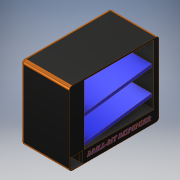
# Autodesk Inventor part: OUTER CASE
Saved by Autodesk Inventor 2019 (Build 230136000, 136)
## iProperties
Created: 2020-03-10
Part Number: OUTER CASE
Material: Gold
Document SubType Name: Modeling
Designer: Hp
Density: 19.3 g/cm^3
Appearance: Metal 1600F Hot
Author: Hp
Autodesk Inventor part; units mm, degrees
ref_plane "YZ Plane" through (0, 0, 0) normal (1, 0, 0) x (0, 1, 0)
ref_plane "XZ Plane" through (0, 0, 0) normal (0, 1, 0) x (-1, 0, 0)
ref_plane "XY Plane" through (0, 0, 0) normal (0, 0, 1) x (1, 0, 0)
sketch "Sketch1" plane through (0, 0, 0) normal (1, 0, 0) x (0, 1, 0)
  line L0 (17.9465, 50) -> (-182.0535, 50)
  line L1 (-182.0535, 50) -> (-182.0535, -300)
  line L2 (-182.0535, -300) -> (17.9465, -300)
  line L3 (17.9465, -300) -> (17.9465, 50)
  point P0 (0, 0)
  dimension "d0" = 200
  dimension "d1" = 350
  constraints: 8 end point, 2 parallel, 1 horizontal, 1 perpendicular
  measures "d0" distance of L2.end L1.end
  measures "d1" distance of L1.end L0.end
extrude "Extrusion1" add sketch "Sketch1" along normal blind 5
sketch "Sketch2" plane through (5, 0, 0) normal (1, 0, 0) x (0, 0, -1)
  circle A0 centre (35, -35.893) radius 14
  line L0 (-50, 17.9465) -> (-50, -182.0535) projected
  line L1 (132.0128, -157.8668) -> (156.8147, -157.8668)
  circle A1 centre (80, -35.893) radius 14
  circle A2 centre (125, -35.893) radius 14
  circle A3 centre (170, -35.893) radius 14
  circle A4 centre (215, -35.893) radius 14
  point P0 (0, 0)
  dimension "d4" = 28
  dimension "d5" = 85
  dimension "d8" = 45
  constraints: 5 centre point, 2 end point, 2 horizontal, 9 other
  measures "d4" diameter of A0
  measures "d8" distance of A0.centre A1.centre
extrude "Extrusion2" cut sketch "Sketch2" against normal blind 1
sketch "Sketch4" plane through (5, 0, 0) normal (1, 0, 0) x (0, 0, -1)
  line L0 (-50, 17.9465) -> (-50, -182.0535) projected
  line L1 (-50, -182.0535) -> (300, -182.0535) projected
  line L2 (-50, 17.9465) -> (0, 17.9465)
  line L3 (0, 17.9465) -> (0, -182.0535)
  line L4 (0, -182.0535) -> (-50, -182.0535)
  line L5 (-50, -182.0535) -> (-50, 17.9465)
  point P0 (0, 0)
  dimension "d17" = 50
  constraints: 8 end point, 2 parallel, 1 horizontal, 1 perpendicular, 1 point on line, 1 other
extrude "Extrusion3" add sketch "Sketch4" along normal blind 150
sketch "Sketch5" plane through (5, 0, 0) normal (1, 0, 0) x (0, 0, -1)
  circle A0 centre (35, -122.0535) radius 14
  line L0 (0, -182.0535) -> (300, -182.0535) projected
  circle A1 centre (80, -122.0535) radius 14
  circle A2 centre (125, -122.0535) radius 14
  circle A3 centre (170, -122.0535) radius 14
  circle A4 centre (215, -122.0535) radius 14
  point P0 (0, 0)
  dimension "d18" = 28
  dimension "d19" = 60
  dimension "d22" = 45
  constraints: 5 centre point, 1 horizontal, 8 other
  measures "d18" diameter of A0
  measures "d19" distance from line of L0 A0.centre
  measures "d22" distance of A0.centre A1.centre
extrude "Extrusion4" cut sketch "Sketch5" against normal blind 2
sketch "Sketch6" plane through (5, 0, 0) normal (1, 0, 0) x (0, 0, -1)
  line L0 (0, -182.0535) -> (300, -182.0535) projected
  line L1 (299.7409, 17.9465) -> (246.5216, 17.9465)
  line L2 (246.5216, 17.9465) -> (246.5216, -182.0535)
  line L3 (246.5216, -182.0535) -> (299.7409, -182.0535)
  line L4 (299.7409, -182.0535) -> (299.7409, 17.9465)
  point P0 (0, 0)
  dimension "d29" = 200
  constraints: 8 end point, 2 parallel, 1 horizontal, 1 perpendicular, 1 point on line
  measures "d29" distance of L3.end L1.start
extrude "Extrusion5" cut sketch "Sketch6" against normal blind 20
sketch "Sketch7" plane through (5, 0, 0) normal (1, 0, 0) x (0, 0, -1)
  line L0 (290.724, 51.1324) -> (325.2992, 51.1324)
  line L1 (325.2992, 51.1324) -> (325.2992, -191.8681)
  line L2 (325.2992, -191.8681) -> (290.724, -191.8681)
  line L3 (290.724, -191.8681) -> (290.724, 51.1324)
  point P0 (0, 0)
  constraints: 8 end point, 2 parallel, 1 horizontal, 1 perpendicular
extrude "Extrusion6" cut sketch "Sketch7" against normal blind 20
sketch "Sketch8" plane through (5, 0, 0) normal (1, 0, 0) x (0, 0, -1)
  line L0 (0, -182.0535) -> (246.5216, -182.0535) projected
  line L1 (246.8963, 18.505) -> (231.8963, 18.505)
  line L2 (231.8963, 18.505) -> (231.8963, -182.0535)
  line L3 (231.8963, -182.0535) -> (246.8963, -182.0535)
  line L4 (246.8963, -182.0535) -> (246.8963, 18.505)
  point P0 (0, 0)
  dimension "d34" = 15
  constraints: 8 end point, 2 parallel, 1 horizontal, 1 perpendicular, 1 point on line
  measures "d34" distance of L3.end L2.end
extrude "Extrusion7" add sketch "Sketch8" along normal blind 150
sketch "Sketch9" plane through (5, -182.0535, 0) normal (0, 0, -1) x (-1, 0, 0)
  point P0 (5, 182.0535)
sketch "Sketch10" plane through (5, 0, 0) normal (1, 0, 0) x (0, 0, -1)
  line L0 (0, -182.0535) -> (0, 17.9465) projected
  line L1 (0, -85.1802) -> (231.8963, -53.9271)
  line L2 (231.8963, -182.0535) -> (231.8963, 17.9465) projected
  line L3 (231.8963, -53.9271) -> (231.8963, -63.9271)
  line L4 (0, -85.1802) -> (0, -95.1802)
  line L5 (0, -95.1802) -> (231.8963, -63.9271)
  line L6 (0, -170.1802) -> (231.8963, -138.9271)
  line L7 (0, -180.1802) -> (231.8963, -148.9271)
  line L8 (0, -170.1802) -> (0, -180.1802)
  line L9 (231.8963, -138.9271) -> (231.8963, -148.9271)
  point P0 (0, 0)
  dimension "d37" = 10
  dimension "d38" = 10
  dimension "d41" = 85
  constraints: 16 end point, 4 point on line, 1 vertical, 8 other
  measures "d37" distance of L1.end L3.end
  measures "d38" distance of L1.start L4.end
  measures "d41" distance of L1.start L6.start
extrude "Extrusion8" add sketch "Sketch10" along normal blind 150 contours L0 L6 L2 L7 | L0 L1 L2 L5
sketch "Sketch11" plane through (0, -182.0535, 50) normal (0, -1, 0) x (1, 0, 0)
  line L0 (150.9028, -4.3641) -> (4.8678, -4.3641)
  line L1 (4.8678, -4.3641) -> (4.8678, -45.7406)
  line L2 (4.8678, -45.7406) -> (150.9028, -45.7406)
  line L3 (150.9028, -45.7406) -> (150.9028, -4.3641)
  point P0 (0, -50)
  constraints: 8 end point, 2 parallel, 1 horizontal, 1 perpendicular
extrude "Extrusion9" cut sketch "Sketch11" against normal blind 190
sketch "Sketch12" plane through (155, 17.9465, 0) normal (0, 0, -1) x (-1, 0, 0)
  line L0 (150, -103.1268) -> (150, -71.8736) projected
  line L1 (150, -103.1268) -> (0, -103.1268)
  line L2 (0, -103.1268) -> (0, -83.1268)
  line L3 (0, -83.1268) -> (150, -83.1268)
  line L4 (150, -83.1268) -> (150, -103.1268)
  line L5 (0, -103.1268) -> (0, 0) projected
  line L6 (150, -188.1268) -> (0, -188.1268)
  line L7 (0, -188.1268) -> (0, -168.1268)
  line L8 (0, -168.1268) -> (150, -168.1268)
  line L9 (150, -168.1268) -> (150, -188.1268)
  point P0 (155, -17.9465)
  dimension "d50" = 20
  dimension "d51" = 0
  dimension "d54" = 85
  constraints: 16 end point, 2 parallel, 1 collinear, 1 horizontal, 1 perpendicular, 1 vertical, 7 other
  measures "d50" distance between parallel lines of L1 L3
  measures "d51" distance between parallel lines of L5 L2
  measures "d54" distance of L2.end L7.end
extrude "Extrusion10" cut sketch "Sketch12" against normal blind 7
fillet "Fillet1" radius 5 2 edges at (77.9514, -85.1802, 4.2594) (77.9514, -170.1802, 4.2594)
sketch "Sketch13" plane through (0, -182.0535, 50) normal (0, -1, 0) x (1, 0, 0)
  line L0 (0, 0) -> (155, 0) projected
  line L1 (0, -296.5216) -> (0, 0) projected
  line L2 (155, 0) -> (0, 0)
  line L3 (0, 0) -> (0, -296.5216)
  line L4 (0, -296.5216) -> (155, -296.5216)
  line L5 (155, -296.5216) -> (155, 0)
  line L6 (4.8678, -4.3641) -> (150.9028, -4.3641) projected
  line L7 (5, -50) -> (5, -45.7406) projected
  line L8 (150.9028, -4.3641) -> (5, -4.3641)
  line L9 (5, -4.3641) -> (5, -45.7406)
  line L10 (5, -45.7406) -> (150.9028, -45.7406)
  line L11 (150.9028, -45.7406) -> (150.9028, -4.3641)
  point P0 (0, -50)
  constraints: 16 end point, 4 parallel, 2 horizontal, 2 perpendicular
extrude "Extrusion11" add sketch "Sketch13" along normal blind 40
sketch "Sketch14" plane through (0, 17.9465, 50) normal (0, 1, 0) x (1, 0, 0)
  line L0 (0, 296.5216) -> (155, 296.5216) projected
  line L1 (0, 0) -> (155, 0)
  line L2 (155, 0) -> (155, 296.5216)
  line L3 (155, 296.5216) -> (0, 296.5216)
  line L4 (0, 296.5216) -> (0, 0)
  point P0 (0, 50)
  constraints: 8 end point, 2 parallel, 1 horizontal, 1 perpendicular
extrude "Extrusion12" add sketch "Sketch14" along normal blind 5
sketch "Sketch15" plane through (155, 18.505, -246.5216) normal (0, 0, -1) x (-1, 0, 0)
  line L0 (155, -240.5585) -> (0, -240.5585) projected
  line L1 (0, -240.5585) -> (155, -240.5585)
  line L2 (155, -240.5585) -> (155, 4.4415)
  line L3 (155, 4.4415) -> (0, 4.4415)
  line L4 (0, 4.4415) -> (0, -240.5585)
  line L5 (0, 4.4415) -> (155, 4.4415) projected
  point P0 (155, -18.505)
  dimension "d66" = 0
  constraints: 8 end point, 2 parallel, 1 horizontal, 1 perpendicular
  measures "d66" distance between parallel lines of L5 L3
extrude "Extrusion13" add sketch "Sketch15" along normal blind 2
sketch "Sketch16" plane through (155, 0, 0) normal (1, 0, 0) x (0, 0, -1)
  line L0 (-50, -222.0535) -> (-50, 22.9465) projected
  line L1 (-50, -222.0535) -> (248.5216, -222.0535) projected
  line L2 (-50, 22.9465) -> (248.5216, 22.9465)
  line L3 (248.5216, 22.9465) -> (248.5216, -222.0535)
  line L4 (248.5216, -222.0535) -> (-50, -222.0535)
  line L5 (-50, -222.0535) -> (-50, 22.9465)
  line L6 (0, 17.9465) -> (0, -65.1802) projected
  line L7 (231.8963, -182.0535) -> (0, -182.0535) projected
  line L8 (0, 17.9465) -> (231.8963, 17.9465)
  line L9 (231.8963, 17.9465) -> (231.8963, -182.0535)
  line L10 (231.8963, -182.0535) -> (0, -182.0535)
  line L11 (0, -182.0535) -> (0, 17.9465)
  point P0 (0, 0)
  constraints: 16 end point, 4 parallel, 2 horizontal, 2 perpendicular
extrude "Extrusion14" add sketch "Sketch16" along normal blind 7
sketch "Sketch17" plane through (162, 0, 0) normal (1, 0, 0) x (0, 0, -1)
  line L0 (-50, -222.0535) -> (248.5216, -222.0535) projected
  line L1 (-45.6359, -182.0535) -> (-45.6359, 7.9465) projected
  line L2 (-4.5693, -222.0535) -> (-45.6359, -222.0535)
  line L3 (-45.6359, -222.0535) -> (-45.6359, -182.0535)
  line L4 (-45.6359, -182.0535) -> (-4.5693, -182.0535)
  line L5 (-4.5693, -182.0535) -> (-4.5693, -222.0535)
  point P0 (0, 0)
  constraints: 8 end point, 2 parallel, 1 horizontal, 1 perpendicular, 1 point on line
extrude "Extrusion15" cut sketch "Sketch17" against normal blind 50
sketch "Sketch18" plane through (0, -222.0535, 50) normal (0, -1, 0) x (1, 0, 0)
  line L0 (162, -298.5216) -> (162, 0) projected
  line L1 (0, 0) -> (162, 0)
  line L2 (162, 0) -> (162, -298.5216)
  line L3 (162, -298.5216) -> (0, -298.5216)
  line L4 (0, -298.5216) -> (0, 0)
  point P0 (0, -50)
  constraints: 8 end point, 2 parallel, 1 horizontal, 1 perpendicular
extrude "Extrusion16" add sketch "Sketch18" against normal blind 2
fillet "Fillet2" radius 10 8 edges at (81, 22.9465, 50) (0, -99.5535, 50) (0, 22.9465, -99.2608) (81, -222.0535, 50) (81, 22.9465, -248.5216) (81, -222.0535, -248.5216) (0, -99.5535, -248.5216) (0, -222.0535, -99.2608)
sketch "Sketch19" plane through (162, 0, 0) normal (1, 0, 0) x (0, 0, -1)
  line L0 (9.1393, -193.2307) -> (248.0665, -193.2307) construction
  line L1 (248.0665, -193.2307) -> (248.0665, -225.8711) construction
  line L2 (248.0665, -225.8711) -> (9.1393, -225.8711) construction
  line L3 (9.1393, -225.8711) -> (9.1393, -193.2307) construction
  line L4 (8.4277, -206.5281) -> (8.5445, -206.1776)
  spline S0 degree 2 poles (8.5445, -206.1776) (9.4792, -206.1776) (10.4457, -205.4023) (10.7643, -204.3296) knots 0 0 0 1 2 2 2
  line L5 (10.7643, -204.3296) -> (13.1221, -196.1302)
  spline S1 degree 2 poles (13.1221, -196.1302) (13.3452, -195.3231) (13.3452, -194.8132) knots 0 0 0 1 1 1
  spline S2 degree 2 poles (13.3452, -194.8132) (13.3452, -194.3672) (12.8141, -193.9423) (11.7096, -193.8786) knots 0 0 0 1 2 2 2
  line L6 (11.7096, -193.8786) -> (11.8264, -193.5281)
  line L7 (11.8264, -193.5281) -> (16.2765, -193.5281)
  spline S3 degree 2 poles (16.2765, -193.5281) (19.7921, -193.5281) (22.904, -196.3745) (22.904, -198.9448) knots 0 0 0 1 2 2 2
  spline S4 degree 2 poles (22.904, -198.9448) (22.904, -200.761) (22.1818, -201.9824) knots 0 0 0 1 1 1
  spline S5 degree 2 poles (22.1818, -201.9824) (20.7798, -204.3827) (16.9032, -206.5281) (13.8656, -206.5281) knots 0 0 0 1 2 2 2
  line L8 (13.8656, -206.5281) -> (8.4277, -206.5281)
  line L9 (16.5314, -194.2928) -> (13.6957, -204.149)
  spline S6 degree 2 poles (13.6957, -204.149) (13.4939, -204.8394) (13.4939, -205.1368) knots 0 0 0 1 1 1
  spline S7 degree 2 poles (13.4939, -205.1368) (13.4939, -205.4023) (13.7063, -205.5616) knots 0 0 0 1 1 1
  spline S8 degree 2 poles (13.7063, -205.5616) (14.0037, -205.7847) (14.5666, -205.7847) knots 0 0 0 1 1 1
  spline S9 degree 2 poles (14.5666, -205.7847) (15.9261, -205.7847) (16.9881, -204.9456) knots 0 0 0 1 1 1
  spline S10 degree 2 poles (16.9881, -204.9456) (18.3582, -203.8516) (19.7921, -200.1874) (19.7921, -198.3925) knots 0 0 0 1 2 2 2
  spline S11 degree 2 poles (19.7921, -198.3925) (19.7921, -197.0861) (18.953, -195.1425) (18.0821, -194.6433) knots 0 0 0 1 2 2 2
  spline S12 degree 2 poles (18.0821, -194.6433) (17.4767, -194.2928) (16.5314, -194.2928) knots 0 0 0 1 1 1
  line L10 (28.9367, -200.1768) -> (27.8109, -204.1172)
  spline S13 degree 2 poles (27.8109, -204.1172) (27.556, -204.9562) (27.556, -205.3492) knots 0 0 0 1 1 1
  spline S14 degree 2 poles (27.556, -205.3492) (27.556, -205.7209) (28.1507, -206.1564) (29.096, -206.1776) knots 0 0 0 1 2 2 2
  line L11 (29.096, -206.1776) -> (28.9579, -206.5281)
  line L12 (28.9579, -206.5281) -> (22.7022, -206.5281)
  line L13 (22.7022, -206.5281) -> (22.8084, -206.1776)
  spline S15 degree 2 poles (22.8084, -206.1776) (23.7537, -206.1776) (24.6246, -205.4448) (24.9857, -204.1809) knots 0 0 0 1 2 2 2
  line L14 (24.9857, -204.1809) -> (27.386, -195.8329)
  spline S16 degree 2 poles (27.386, -195.8329) (27.5878, -195.1319) (27.5878, -194.7283) knots 0 0 0 1 1 1
  spline S17 degree 2 poles (27.5878, -194.7283) (27.5878, -194.3459) (27.0886, -193.9423) (26.1752, -193.8786) knots 0 0 0 1 2 2 2
  line L15 (26.1752, -193.8786) -> (26.2708, -193.5281)
  line L16 (26.2708, -193.5281) -> (31.6769, -193.5281)
  spline S18 degree 2 poles (31.6769, -193.5281) (33.9922, -193.5281) (35.8721, -195.1319) (35.8721, -196.4064) knots 0 0 0 1 2 2 2
  spline S19 degree 2 poles (35.8721, -196.4064) (35.8721, -197.734) (34.7676, -198.8067) knots 0 0 0 1 1 1
  spline S20 degree 2 poles (34.7676, -198.8067) (34.0772, -199.4758) (32.3035, -199.9644) knots 0 0 0 1 1 1
  line L17 (32.3035, -199.9644) -> (33.4612, -203.9048)
  spline S21 degree 2 poles (33.4612, -203.9048) (33.9391, -205.4979) (34.6401, -206.1458) (35.4473, -206.1776) knots 0 0 0 1 2 2 2
  line L18 (35.4473, -206.1776) -> (35.4473, -206.5281)
  line L19 (35.4473, -206.5281) -> (31.4007, -206.5281)
  line L20 (31.4007, -206.5281) -> (29.5739, -200.1768)
  line L21 (29.5739, -200.1768) -> (29.2553, -200.1981)
  spline S22 degree 2 poles (29.2553, -200.1981) (29.1491, -200.1981) (28.9367, -200.1768) knots 0 0 0 1 1 1
  spline S23 degree 2 poles (29.096, -199.6033) (29.4252, -199.6245) (29.6483, -199.6245) knots 0 0 0 1 1 1
  spline S24 degree 2 poles (29.6483, -199.6245) (31.029, -199.6245) (32.8133, -197.7021) (32.8133, -196.1515) knots 0 0 0 1 2 2 2
  spline S25 degree 2 poles (32.8133, -196.1515) (32.8133, -195.2275) (31.8574, -194.2716) (31.0821, -194.2716) knots 0 0 0 1 2 2 2
  spline S26 degree 2 poles (31.0821, -194.2716) (30.8909, -194.2716) (30.6254, -194.2822) knots 0 0 0 1 1 1
  line L22 (30.6254, -194.2822) -> (29.096, -199.6033)
  line L23 (39.1115, -193.8786) -> (39.2177, -193.5281)
  line L24 (39.2177, -193.5281) -> (45.5796, -193.5281)
  line L25 (45.5796, -193.5281) -> (45.4522, -193.8786)
  spline S27 degree 2 poles (45.4522, -193.8786) (44.5919, -193.8786) (43.6785, -194.6433) (43.328, -195.8647) knots 0 0 0 1 2 2 2
  line L26 (43.328, -195.8647) -> (40.9596, -204.1915)
  spline S28 degree 2 poles (40.9596, -204.1915) (40.694, -205.0731) (40.694, -205.3704) knots 0 0 0 1 1 1
  spline S29 degree 2 poles (40.694, -205.3704) (40.694, -205.7209) (40.9702, -205.9121) knots 0 0 0 1 1 1
  spline S30 degree 2 poles (40.9702, -205.9121) (41.31, -206.1564) (42.2659, -206.1776) knots 0 0 0 1 1 1
  line L27 (42.2659, -206.1776) -> (42.1703, -206.5281)
  line L28 (42.1703, -206.5281) -> (35.7234, -206.5281)
  line L29 (35.7234, -206.5281) -> (35.8296, -206.1776)
  spline S31 degree 2 poles (35.8296, -206.1776) (36.7962, -206.1776) (37.6989, -205.4342) (38.06, -204.1915) knots 0 0 0 1 2 2 2
  line L30 (38.06, -204.1915) -> (40.4497, -195.8647)
  spline S32 degree 2 poles (40.4497, -195.8647) (40.6728, -195.1) (40.6728, -194.707) knots 0 0 0 1 1 1
  spline S33 degree 2 poles (40.6728, -194.707) (40.6728, -194.3459) (40.1311, -193.9423) (39.1115, -193.8786) knots 0 0 0 1 2 2 2
  line L31 (53.8109, -206.5281) -> (43.4342, -206.5281)
  line L32 (43.4342, -206.5281) -> (43.5404, -206.1776)
  spline S34 degree 2 poles (43.5404, -206.1776) (44.4645, -206.1776) (45.3247, -205.4554) (45.6859, -204.2021) knots 0 0 0 1 2 2 2
  line L33 (45.6859, -204.2021) -> (48.0756, -195.8435)
  spline S35 degree 2 poles (48.0756, -195.8435) (48.2774, -195.1531) (48.2774, -194.7601) knots 0 0 0 1 1 1
  spline S36 degree 2 poles (48.2774, -194.7601) (48.2774, -194.3778) (47.7038, -193.9211) (46.8648, -193.8786) knots 0 0 0 1 2 2 2
  line L34 (46.8648, -193.8786) -> (46.971, -193.5281)
  line L35 (46.971, -193.5281) -> (53.2161, -193.5281)
  line L36 (53.2161, -193.5281) -> (53.1099, -193.8786)
  spline S37 degree 2 poles (53.1099, -193.8786) (52.2071, -193.8999) (51.3149, -194.6646) (50.9751, -195.8435) knots 0 0 0 1 2 2 2
  line L37 (50.9751, -195.8435) -> (48.7765, -203.4799)
  spline S38 degree 2 poles (48.7765, -203.4799) (48.3517, -204.9456) (48.3517, -205.2536) knots 0 0 0 1 1 1
  spline S39 degree 2 poles (48.3517, -205.2536) (48.3517, -205.4448) (48.7872, -205.7847) (49.2651, -205.7847) knots 0 0 0 1 2 2 2
  spline S40 degree 2 poles (49.2651, -205.7847) (50.8582, -205.7847) (53.8215, -204.3296) (54.8411, -202.8851) knots 0 0 0 1 2 2 2
  line L38 (54.8411, -202.8851) -> (55.2447, -202.8851)
  line L39 (55.2447, -202.8851) -> (53.8109, -206.5281)
  line L40 (65.8019, -206.5281) -> (55.4252, -206.5281)
  line L41 (55.4252, -206.5281) -> (55.5314, -206.1776)
  spline S41 degree 2 poles (55.5314, -206.1776) (56.4555, -206.1776) (57.3158, -205.4554) (57.6769, -204.2021) knots 0 0 0 1 2 2 2
  line L42 (57.6769, -204.2021) -> (60.0666, -195.8435)
  spline S42 degree 2 poles (60.0666, -195.8435) (60.2684, -195.1531) (60.2684, -194.7601) knots 0 0 0 1 1 1
  spline S43 degree 2 poles (60.2684, -194.7601) (60.2684, -194.3778) (59.6948, -193.9211) (58.8558, -193.8786) knots 0 0 0 1 2 2 2
  line L43 (58.8558, -193.8786) -> (58.962, -193.5281)
  line L44 (58.962, -193.5281) -> (65.2071, -193.5281)
  line L45 (65.2071, -193.5281) -> (65.1009, -193.8786)
  spline S44 degree 2 poles (65.1009, -193.8786) (64.1981, -193.8999) (63.306, -194.6646) (62.9661, -195.8435) knots 0 0 0 1 2 2 2
  line L46 (62.9661, -195.8435) -> (60.7676, -203.4799)
  spline S45 degree 2 poles (60.7676, -203.4799) (60.3427, -204.9456) (60.3427, -205.2536) knots 0 0 0 1 1 1
  spline S46 degree 2 poles (60.3427, -205.2536) (60.3427, -205.4448) (60.7782, -205.7847) (61.2561, -205.7847) knots 0 0 0 1 2 2 2
  spline S47 degree 2 poles (61.2561, -205.7847) (62.8493, -205.7847) (65.8125, -204.3296) (66.8321, -202.8851) knots 0 0 0 1 2 2 2
  line L47 (66.8321, -202.8851) -> (67.2357, -202.8851)
  line L48 (67.2357, -202.8851) -> (65.8019, -206.5281)
  line L49 (68.7863, -201.2283) -> (74.3517, -201.2283)
  line L50 (74.3517, -201.2283) -> (73.7676, -203.225)
  line L51 (73.7676, -203.225) -> (68.1597, -203.225)
  line L52 (68.1597, -203.225) -> (68.7863, -201.2283)
  line L53 (77.5911, -193.5281) -> (82.7422, -193.5281)
  spline S48 degree 2 poles (82.7422, -193.5281) (84.4628, -193.5281) (85.2063, -193.7087) knots 0 0 0 1 1 1
  spline S49 degree 2 poles (85.2063, -193.7087) (86.1834, -193.9423) (87.2455, -195.2699) (87.2455, -196.109) knots 0 0 0 1 2 2 2
  spline S50 degree 2 poles (87.2455, -196.109) (87.2455, -196.7994) (86.3852, -198.2438) (84.6859, -199.1678) (82.9334, -199.5608) knots 0 0 0 1 2 3 3 3
  spline S51 degree 2 poles (82.9334, -199.5608) (84.7708, -200.0706) (86.194, -201.6637) (86.194, -202.7152) knots 0 0 0 1 2 2 2
  spline S52 degree 2 poles (86.194, -202.7152) (86.194, -203.703) (84.8133, -205.636) (82.5298, -206.5281) (79.4922, -206.5281) knots 0 0 0 1 2 3 3 3
  line L54 (79.4922, -206.5281) -> (74.0862, -206.5281)
  line L55 (74.0862, -206.5281) -> (74.2136, -206.1776)
  spline S53 degree 2 poles (74.2136, -206.1776) (74.9996, -206.1776) (75.6793, -205.8909) (76.0829, -205.2855) (76.3697, -204.319) knots 0 0 0 1 2 3 3 3
  line L56 (76.3697, -204.319) -> (78.6532, -196.3214)
  spline S54 degree 2 poles (78.6532, -196.3214) (79.0143, -195.1106) (79.0143, -194.6964) knots 0 0 0 1 1 1
  spline S55 degree 2 poles (79.0143, -194.6964) (79.0143, -194.3566) (78.4514, -193.9211) (77.4955, -193.8786) knots 0 0 0 1 2 2 2
  line L57 (77.4955, -193.8786) -> (77.5911, -193.5281)
  line L58 (80.3313, -199.9856) -> (78.685, -205.7634)
  spline S56 degree 2 poles (78.685, -205.7634) (79.1524, -205.7847) (79.386, -205.7847) knots 0 0 0 1 1 1
  spline S57 degree 2 poles (79.386, -205.7847) (81.489, -205.7847) (83.1352, -203.3949) (83.1352, -202.0355) knots 0 0 0 1 2 2 2
  spline S58 degree 2 poles (83.1352, -202.0355) (83.1352, -201.3876) (82.5086, -200.3786) (81.5102, -199.9856) (80.3313, -199.9856) knots 0 0 0 1 2 3 3 3
  spline S59 degree 2 poles (80.5437, -199.2634) (81.8182, -199.2422) (83.2945, -198.4562) (84.1867, -196.6719) (84.1867, -195.8753) knots 0 0 0 1 2 3 3 3
  spline S60 degree 2 poles (84.1867, -195.8753) (84.1867, -195.1213) (83.2733, -194.1866) (82.4979, -194.2079) knots 0 0 0 1 2 2 2
  line L59 (82.4979, -194.2079) -> (81.9881, -194.2291)
  line L60 (81.9881, -194.2291) -> (80.5437, -199.2634)
  line L61 (90.3787, -193.8786) -> (90.4849, -193.5281)
  line L62 (90.4849, -193.5281) -> (96.8468, -193.5281)
  line L63 (96.8468, -193.5281) -> (96.7194, -193.8786)
  spline S61 degree 2 poles (96.7194, -193.8786) (95.8591, -193.8786) (94.9457, -194.6433) (94.5952, -195.8647) knots 0 0 0 1 2 2 2
  line L64 (94.5952, -195.8647) -> (92.2267, -204.1915)
  spline S62 degree 2 poles (92.2267, -204.1915) (91.9612, -205.0731) (91.9612, -205.3704) knots 0 0 0 1 1 1
  spline S63 degree 2 poles (91.9612, -205.3704) (91.9612, -205.7209) (92.2373, -205.9121) knots 0 0 0 1 1 1
  spline S64 degree 2 poles (92.2373, -205.9121) (92.5772, -206.1564) (93.5331, -206.1776) knots 0 0 0 1 1 1
  line L65 (93.5331, -206.1776) -> (93.4375, -206.5281)
  line L66 (93.4375, -206.5281) -> (86.9906, -206.5281)
  line L67 (86.9906, -206.5281) -> (87.0968, -206.1776)
  spline S65 degree 2 poles (87.0968, -206.1776) (88.0633, -206.1776) (88.9661, -205.4342) (89.3272, -204.1915) knots 0 0 0 1 2 2 2
  line L68 (89.3272, -204.1915) -> (91.7169, -195.8647)
  spline S66 degree 2 poles (91.7169, -195.8647) (91.9399, -195.1) (91.9399, -194.707) knots 0 0 0 1 1 1
  spline S67 degree 2 poles (91.9399, -194.707) (91.9399, -194.3459) (91.3983, -193.9423) (90.3787, -193.8786) knots 0 0 0 1 2 2 2
  line L69 (98.4824, -193.5281) -> (108.9334, -193.5281)
  line L70 (108.9334, -193.5281) -> (107.9457, -197.033)
  line L71 (107.9457, -197.033) -> (107.6058, -197.033)
  spline S68 degree 2 poles (107.6058, -197.033) (107.627, -196.7569) (107.627, -196.5445) knots 0 0 0 1 1 1
  spline S69 degree 2 poles (107.627, -196.5445) (107.627, -195.5461) (106.4056, -194.4415) (104.9612, -194.3672) knots 0 0 0 1 2 2 2
  line L72 (104.9612, -194.3672) -> (102.1573, -204.1597)
  spline S70 degree 2 poles (102.1573, -204.1597) (101.9236, -204.9668) (101.9236, -205.3598) knots 0 0 0 1 1 1
  spline S71 degree 2 poles (101.9236, -205.3598) (101.9236, -205.7316) (102.5184, -206.1564) (103.4212, -206.1776) knots 0 0 0 1 2 2 2
  line L73 (103.4212, -206.1776) -> (103.3362, -206.5281)
  line L74 (103.3362, -206.5281) -> (96.8893, -206.5281)
  line L75 (96.8893, -206.5281) -> (97.0061, -206.1776)
  spline S72 degree 2 poles (97.0061, -206.1776) (97.9939, -206.1776) (98.8966, -205.4342) (99.2684, -204.149) knots 0 0 0 1 2 2 2
  line L76 (99.2684, -204.149) -> (102.0723, -194.3672)
  spline S73 degree 2 poles (102.0723, -194.3672) (100.6172, -194.4203) (98.6417, -195.6204) (97.8239, -197.033) knots 0 0 0 1 2 2 2
  line L77 (97.8239, -197.033) -> (97.4522, -197.033)
  line L78 (97.4522, -197.033) -> (98.4824, -193.5281)
  line L79 (111.5143, -206.5281) -> (111.6311, -206.1776)
  spline S74 degree 2 poles (111.6311, -206.1776) (112.5658, -206.1776) (113.5323, -205.4023) (113.8509, -204.3296) knots 0 0 0 1 2 2 2
  line L80 (113.8509, -204.3296) -> (116.2087, -196.1302)
  spline S75 degree 2 poles (116.2087, -196.1302) (116.4318, -195.3231) (116.4318, -194.8132) knots 0 0 0 1 1 1
  spline S76 degree 2 poles (116.4318, -194.8132) (116.4318, -194.3672) (115.9007, -193.9423) (114.7961, -193.8786) knots 0 0 0 1 2 2 2
  line L81 (114.7961, -193.8786) -> (114.913, -193.5281)
  line L82 (114.913, -193.5281) -> (119.3631, -193.5281)
  spline S77 degree 2 poles (119.3631, -193.5281) (122.8787, -193.5281) (125.9906, -196.3745) (125.9906, -198.9448) knots 0 0 0 1 2 2 2
  spline S78 degree 2 poles (125.9906, -198.9448) (125.9906, -200.761) (125.2684, -201.9824) knots 0 0 0 1 1 1
  spline S79 degree 2 poles (125.2684, -201.9824) (123.8664, -204.3827) (119.9898, -206.5281) (116.9522, -206.5281) knots 0 0 0 1 2 2 2
  line L83 (116.9522, -206.5281) -> (111.5143, -206.5281)
  line L84 (119.618, -194.2928) -> (116.7823, -204.149)
  spline S80 degree 2 poles (116.7823, -204.149) (116.5805, -204.8394) (116.5805, -205.1368) knots 0 0 0 1 1 1
  spline S81 degree 2 poles (116.5805, -205.1368) (116.5805, -205.4023) (116.7929, -205.5616) knots 0 0 0 1 1 1
  spline S82 degree 2 poles (116.7929, -205.5616) (117.0903, -205.7847) (117.6532, -205.7847) knots 0 0 0 1 1 1
  spline S83 degree 2 poles (117.6532, -205.7847) (119.0127, -205.7847) (120.0747, -204.9456) knots 0 0 0 1 1 1
  spline S84 degree 2 poles (120.0747, -204.9456) (121.4448, -203.8516) (122.8787, -200.1874) (122.8787, -198.3925) knots 0 0 0 1 2 2 2
  spline S85 degree 2 poles (122.8787, -198.3925) (122.8787, -197.0861) (122.0396, -195.1425) (121.1687, -194.6433) knots 0 0 0 1 2 2 2
  spline S86 degree 2 poles (121.1687, -194.6433) (120.5633, -194.2928) (119.618, -194.2928) knots 0 0 0 1 1 1
  line L85 (129.1025, -193.8786) -> (129.2087, -193.5281)
  line L86 (129.2087, -193.5281) -> (135.5707, -193.5281)
  line L87 (135.5707, -193.5281) -> (135.4432, -193.8786)
  spline S87 degree 2 poles (135.4432, -193.8786) (134.5829, -193.8786) (133.6695, -194.6433) (133.319, -195.8647) knots 0 0 0 1 2 2 2
  line L88 (133.319, -195.8647) -> (130.9506, -204.1915)
  spline S88 degree 2 poles (130.9506, -204.1915) (130.685, -205.0731) (130.685, -205.3704) knots 0 0 0 1 1 1
  spline S89 degree 2 poles (130.685, -205.3704) (130.685, -205.7209) (130.9612, -205.9121) knots 0 0 0 1 1 1
  spline S90 degree 2 poles (130.9612, -205.9121) (131.3011, -206.1564) (132.2569, -206.1776) knots 0 0 0 1 1 1
  line L89 (132.2569, -206.1776) -> (132.1613, -206.5281)
  line L90 (132.1613, -206.5281) -> (125.7145, -206.5281)
  line L91 (125.7145, -206.5281) -> (125.8207, -206.1776)
  spline S91 degree 2 poles (125.8207, -206.1776) (126.7872, -206.1776) (127.6899, -205.4342) (128.0511, -204.1915) knots 0 0 0 1 2 2 2
  line L92 (128.0511, -204.1915) -> (130.4408, -195.8647)
  spline S92 degree 2 poles (130.4408, -195.8647) (130.6638, -195.1) (130.6638, -194.707) knots 0 0 0 1 1 1
  spline S93 degree 2 poles (130.6638, -194.707) (130.6638, -194.3459) (130.1221, -193.9423) (129.1025, -193.8786) knots 0 0 0 1 2 2 2
  line L93 (145.5118, -193.2307) -> (144.4285, -197.6384)
  line L94 (144.4285, -197.6384) -> (144.1099, -197.6384)
  spline S94 degree 2 poles (144.1099, -197.6384) (144.0037, -196.6082) (143.7381, -195.9816) knots 0 0 0 1 1 1
  spline S95 degree 2 poles (143.7381, -195.9816) (143.3345, -195.0788) (141.9963, -194.1016) (141.221, -194.1016) knots 0 0 0 1 2 2 2
  spline S96 degree 2 poles (141.221, -194.1016) (140.4775, -194.1016) (139.3517, -195.2381) (139.3517, -195.9603) knots 0 0 0 1 2 2 2
  spline S97 degree 2 poles (139.3517, -195.9603) (139.3517, -196.6719) (140.127, -198.042) (141.5821, -199.4227) knots 0 0 0 1 2 2 2
  spline S98 degree 2 poles (141.5821, -199.4227) (142.7398, -200.5273) (143.5363, -202.1204) (143.5363, -203.0445) knots 0 0 0 1 2 2 2
  spline S99 degree 2 poles (143.5363, -203.0445) (143.5363, -204.0959) (142.4211, -205.859) (140.3076, -206.8255) (138.9587, -206.8255) knots 0 0 0 1 2 3 3 3
  spline S100 degree 2 poles (138.9587, -206.8255) (138.1409, -206.8255) (135.6344, -206.3369) (135.2202, -206.3369) knots 0 0 0 1 2 2 2
  spline S101 degree 2 poles (135.2202, -206.3369) (134.8909, -206.3369) (134.3811, -206.5387) (133.9988, -206.8255) knots 0 0 0 1 2 2 2
  line L95 (133.9988, -206.8255) -> (133.627, -206.8255)
  line L96 (133.627, -206.8255) -> (134.7741, -201.8655)
  line L97 (134.7741, -201.8655) -> (135.1352, -201.8655)
  spline S102 degree 2 poles (135.1352, -201.8655) (135.252, -203.1719) (136.0592, -204.9987) (137.5674, -206.0289) (138.5233, -206.0289) knots 0 0 0 1 2 3 3 3
  spline S103 degree 2 poles (138.5233, -206.0289) (139.4792, -206.0289) (140.7537, -204.7757) (140.7537, -203.926) knots 0 0 0 1 2 2 2
  spline S104 degree 2 poles (140.7537, -203.926) (140.7537, -203.2144) (140.0314, -201.8868) (137.4718, -199.359) (136.9832, -198.3606) knots 0 0 0 1 2 3 3 3
  spline S105 degree 2 poles (136.9832, -198.3606) (136.6328, -197.6172) (136.6328, -196.7887) knots 0 0 0 1 1 1
  spline S106 degree 2 poles (136.6328, -196.7887) (136.6328, -195.3443) (138.9162, -193.2307) (140.7537, -193.2307) knots 0 0 0 1 2 2 2
  spline S107 degree 2 poles (140.7537, -193.2307) (141.5927, -193.2307) (142.9522, -193.6025) knots 0 0 0 1 1 1
  spline S108 degree 2 poles (142.9522, -193.6025) (143.7488, -193.8255) (144.0674, -193.8255) knots 0 0 0 1 1 1
  spline S109 degree 2 poles (144.0674, -193.8255) (144.3435, -193.8255) (144.7896, -193.5812) (145.087, -193.2307) knots 0 0 0 1 2 2 2
  line L98 (145.087, -193.2307) -> (145.5118, -193.2307)
  line L99 (150.5037, -200.5485) -> (149.4841, -204.1809)
  spline S110 degree 2 poles (149.4841, -204.1809) (149.261, -204.9456) (149.261, -205.2642) knots 0 0 0 1 1 1
  spline S111 degree 2 poles (149.261, -205.2642) (149.261, -205.7103) (149.8345, -206.1564) (150.8542, -206.1776) knots 0 0 0 1 2 2 2
  line L100 (150.8542, -206.1776) -> (150.7267, -206.5281)
  line L101 (150.7267, -206.5281) -> (144.386, -206.5281)
  line L102 (144.386, -206.5281) -> (144.4922, -206.1776)
  spline S112 degree 2 poles (144.4922, -206.1776) (145.2888, -206.167) (145.9685, -205.8696) (146.181, -205.5298) knots 0 0 0 1 2 2 2
  spline S113 degree 2 poles (146.181, -205.5298) (146.3509, -205.3173) (146.6695, -204.1809) knots 0 0 0 1 1 1
  line L103 (146.6695, -204.1809) -> (149.038, -195.9178)
  spline S114 degree 2 poles (149.038, -195.9178) (149.2929, -195.1) (149.2929, -194.7389) knots 0 0 0 1 1 1
  spline S115 degree 2 poles (149.2929, -194.7389) (149.2929, -194.3884) (148.6556, -193.8999) (147.8272, -193.8786) knots 0 0 0 1 2 2 2
  line L104 (147.8272, -193.8786) -> (147.9334, -193.5281)
  line L105 (147.9334, -193.5281) -> (153.1058, -193.5281)
  spline S116 degree 2 poles (153.1058, -193.5281) (155.23, -193.5281) (156.1646, -194.0698) knots 0 0 0 1 1 1
  spline S117 degree 2 poles (156.1646, -194.0698) (157.6091, -194.9088) (157.6091, -196.5976) knots 0 0 0 1 1 1
  spline S118 degree 2 poles (157.6091, -196.5976) (157.6091, -198.2226) (154.7308, -200.7079) (152.288, -200.7079) knots 0 0 0 1 2 2 2
  spline S119 degree 2 poles (152.288, -200.7079) (151.5551, -200.7079) (150.5037, -200.5485) knots 0 0 0 1 1 1
  spline S120 degree 2 poles (150.7161, -199.8157) (151.3321, -199.89) (151.7357, -199.89) knots 0 0 0 1 1 1
  spline S121 degree 2 poles (151.7357, -199.89) (153.0527, -199.89) (154.5502, -197.4791) (154.5502, -196.1621) knots 0 0 0 1 2 2 2
  spline S122 degree 2 poles (154.5502, -196.1621) (154.5502, -195.2699) (153.5731, -194.2822) (152.7128, -194.2822) knots 0 0 0 1 2 2 2
  spline S123 degree 2 poles (152.7128, -194.2822) (152.5323, -194.2822) (152.2667, -194.3034) knots 0 0 0 1 1 1
  line L106 (152.2667, -194.3034) -> (150.7161, -199.8157)
  line L107 (164.3321, -194.2503) -> (162.8983, -199.2847)
  line L108 (162.8983, -199.2847) -> (163.3444, -199.2847)
  spline S124 degree 2 poles (163.3444, -199.2847) (165.0862, -199.2847) (166.6899, -198.3606) (167.2422, -197.1923) knots 0 0 0 1 2 2 2
  line L109 (167.2422, -197.1923) -> (167.5927, -197.1923)
  line L110 (167.5927, -197.1923) -> (166.1483, -202.2585)
  line L111 (166.1483, -202.2585) -> (165.8084, -202.2585)
  spline S125 degree 2 poles (165.8084, -202.2585) (165.8934, -201.7487) (165.8934, -201.4301) knots 0 0 0 1 1 1
  spline S126 degree 2 poles (165.8934, -201.4301) (165.8934, -200.9097) (165.2774, -200.2405) (164.7782, -200.0918) knots 0 0 0 1 2 2 2
  spline S127 degree 2 poles (164.7782, -200.0918) (164.4595, -199.9963) (163.4399, -199.9963) knots 0 0 0 1 1 1
  line L112 (163.4399, -199.9963) -> (162.6965, -199.9963)
  line L113 (162.6965, -199.9963) -> (161.4538, -204.3615)
  spline S128 degree 2 poles (161.4538, -204.3615) (161.2945, -204.935) (161.2945, -205.2111) knots 0 0 0 1 1 1
  spline S129 degree 2 poles (161.2945, -205.2111) (161.2945, -205.4342) (161.4963, -205.5722) knots 0 0 0 1 1 1
  spline S130 degree 2 poles (161.4963, -205.5722) (161.8043, -205.7634) (162.6646, -205.7634) knots 0 0 0 1 1 1
  spline S131 degree 2 poles (162.6646, -205.7634) (164.3002, -205.7634) (167.1997, -204.3721) (168.3468, -202.9595) knots 0 0 0 1 2 2 2
  line L114 (168.3468, -202.9595) -> (168.7398, -202.9595)
  line L115 (168.7398, -202.9595) -> (167.3909, -206.5281)
  line L116 (167.3909, -206.5281) -> (156.3983, -206.5281)
  line L117 (156.3983, -206.5281) -> (156.5151, -206.1776)
  spline S132 degree 2 poles (156.5151, -206.1776) (157.4391, -206.1776) (158.2888, -205.4342) (158.6287, -204.1809) knots 0 0 0 1 2 2 2
  line L118 (158.6287, -204.1809) -> (161.029, -195.801)
  spline S133 degree 2 poles (161.029, -195.801) (161.2308, -195.1106) (161.2308, -194.707) knots 0 0 0 1 1 1
  spline S134 degree 2 poles (161.2308, -194.707) (161.2308, -194.3353) (160.6997, -193.9423) (159.7439, -193.8786) knots 0 0 0 1 2 2 2
  line L119 (159.7439, -193.8786) -> (159.8501, -193.5281)
  line L120 (159.8501, -193.5281) -> (170.3117, -193.5281)
  line L121 (170.3117, -193.5281) -> (169.4726, -196.7781)
  line L122 (169.4726, -196.7781) -> (169.1327, -196.7781)
  spline S135 degree 2 poles (169.1327, -196.7781) (169.0903, -195.8222) (168.8354, -195.4293) knots 0 0 0 1 1 1
  spline S136 degree 2 poles (168.8354, -195.4293) (168.4211, -194.8132) (167.0723, -194.2503) (165.5641, -194.2503) knots 0 0 0 1 2 2 2
  line L123 (165.5641, -194.2503) -> (164.3321, -194.2503)
  line L124 (176.9816, -193.5281) -> (181.0388, -202.216)
  line L125 (181.0388, -202.216) -> (182.8443, -195.8753)
  spline S137 degree 2 poles (182.8443, -195.8753) (182.9824, -195.3655) (182.9824, -194.9619) knots 0 0 0 1 1 1
  spline S138 degree 2 poles (182.9824, -194.9619) (182.9824, -194.4946) (182.377, -193.9211) (181.6442, -193.8786) knots 0 0 0 1 2 2 2
  line L126 (181.6442, -193.8786) -> (181.7504, -193.5281)
  line L127 (181.7504, -193.5281) -> (185.8501, -193.5281)
  line L128 (185.8501, -193.5281) -> (185.7545, -193.8786)
  spline S139 degree 2 poles (185.7545, -193.8786) (184.9685, -193.9317) (183.9383, -194.7177) (183.5878, -195.9072) knots 0 0 0 1 2 2 2
  line L129 (183.5878, -195.9072) -> (180.4971, -206.6768)
  line L130 (180.4971, -206.6768) -> (180.1785, -206.6768)
  line L131 (180.1785, -206.6768) -> (174.9105, -195.5886)
  line L132 (174.9105, -195.5886) -> (172.4252, -204.2234)
  spline S140 degree 2 poles (172.4252, -204.2234) (172.3084, -204.6801) (172.3084, -205.0306) knots 0 0 0 1 1 1
  spline S141 degree 2 poles (172.3084, -205.0306) (172.3084, -205.551) (172.9881, -206.1776) (173.7316, -206.1776) knots 0 0 0 1 2 2 2
  line L133 (173.7316, -206.1776) -> (173.6466, -206.5281)
  line L134 (173.6466, -206.5281) -> (169.4089, -206.5281)
  line L135 (169.4089, -206.5281) -> (169.4939, -206.1776)
  spline S142 degree 2 poles (169.4939, -206.1776) (170.0461, -206.1776) (170.2692, -206.082) knots 0 0 0 1 1 1
  spline S143 degree 2 poles (170.2692, -206.082) (170.6728, -205.9333) (171.4375, -205.0518) (171.6818, -204.234) knots 0 0 0 1 2 2 2
  line L136 (171.6818, -204.234) -> (174.3901, -194.7814)
  spline S144 degree 2 poles (174.3901, -194.7814) (173.9122, -194.2185) (173.2749, -193.8892) (172.627, -193.8786) knots 0 0 0 1 2 2 2
  line L137 (172.627, -193.8786) -> (172.7332, -193.5281)
  line L138 (172.7332, -193.5281) -> (176.9816, -193.5281)
  line L139 (195.6957, -193.2307) -> (194.6123, -197.6384)
  line L140 (194.6123, -197.6384) -> (194.2937, -197.6384)
  spline S145 degree 2 poles (194.2937, -197.6384) (194.1875, -196.6082) (193.922, -195.9816) knots 0 0 0 1 1 1
  spline S146 degree 2 poles (193.922, -195.9816) (193.5184, -195.0788) (192.1801, -194.1016) (191.4048, -194.1016) knots 0 0 0 1 2 2 2
  spline S147 degree 2 poles (191.4048, -194.1016) (190.6613, -194.1016) (189.5355, -195.2381) (189.5355, -195.9603) knots 0 0 0 1 2 2 2
  spline S148 degree 2 poles (189.5355, -195.9603) (189.5355, -196.6719) (190.3109, -198.042) (191.7659, -199.4227) knots 0 0 0 1 2 2 2
  spline S149 degree 2 poles (191.7659, -199.4227) (192.9236, -200.5273) (193.7202, -202.1204) (193.7202, -203.0445) knots 0 0 0 1 2 2 2
  spline S150 degree 2 poles (193.7202, -203.0445) (193.7202, -204.0959) (192.605, -205.859) (190.4914, -206.8255) (189.1426, -206.8255) knots 0 0 0 1 2 3 3 3
  spline S151 degree 2 poles (189.1426, -206.8255) (188.3247, -206.8255) (185.8182, -206.3369) (185.404, -206.3369) knots 0 0 0 1 2 2 2
  spline S152 degree 2 poles (185.404, -206.3369) (185.0747, -206.3369) (184.5649, -206.5387) (184.1826, -206.8255) knots 0 0 0 1 2 2 2
  line L141 (184.1826, -206.8255) -> (183.8109, -206.8255)
  line L142 (183.8109, -206.8255) -> (184.9579, -201.8655)
  line L143 (184.9579, -201.8655) -> (185.319, -201.8655)
  spline S153 degree 2 poles (185.319, -201.8655) (185.4359, -203.1719) (186.243, -204.9987) (187.7512, -206.0289) (188.7071, -206.0289) knots 0 0 0 1 2 3 3 3
  spline S154 degree 2 poles (188.7071, -206.0289) (189.663, -206.0289) (190.9375, -204.7757) (190.9375, -203.926) knots 0 0 0 1 2 2 2
  spline S155 degree 2 poles (190.9375, -203.926) (190.9375, -203.2144) (190.2153, -201.8868) (187.6556, -199.359) (187.1671, -198.3606) knots 0 0 0 1 2 3 3 3
  spline S156 degree 2 poles (187.1671, -198.3606) (186.8166, -197.6172) (186.8166, -196.7887) knots 0 0 0 1 1 1
  spline S157 degree 2 poles (186.8166, -196.7887) (186.8166, -195.3443) (189.1001, -193.2307) (190.9375, -193.2307) knots 0 0 0 1 2 2 2
  spline S158 degree 2 poles (190.9375, -193.2307) (191.7765, -193.2307) (193.136, -193.6025) knots 0 0 0 1 1 1
  spline S159 degree 2 poles (193.136, -193.6025) (193.9326, -193.8255) (194.2512, -193.8255) knots 0 0 0 1 1 1
  spline S160 degree 2 poles (194.2512, -193.8255) (194.5274, -193.8255) (194.9734, -193.5812) (195.2708, -193.2307) knots 0 0 0 1 2 2 2
  line L144 (195.2708, -193.2307) -> (195.6957, -193.2307)
  line L145 (202.5249, -194.2503) -> (201.0911, -199.2847)
  line L146 (201.0911, -199.2847) -> (201.5372, -199.2847)
  spline S161 degree 2 poles (201.5372, -199.2847) (203.279, -199.2847) (204.8827, -198.3606) (205.435, -197.1923) knots 0 0 0 1 2 2 2
  line L147 (205.435, -197.1923) -> (205.7855, -197.1923)
  line L148 (205.7855, -197.1923) -> (204.3411, -202.2585)
  line L149 (204.3411, -202.2585) -> (204.0012, -202.2585)
  spline S162 degree 2 poles (204.0012, -202.2585) (204.0862, -201.7487) (204.0862, -201.4301) knots 0 0 0 1 1 1
  spline S163 degree 2 poles (204.0862, -201.4301) (204.0862, -200.9097) (203.4702, -200.2405) (202.971, -200.0918) knots 0 0 0 1 2 2 2
  spline S164 degree 2 poles (202.971, -200.0918) (202.6524, -199.9963) (201.6327, -199.9963) knots 0 0 0 1 1 1
  line L150 (201.6327, -199.9963) -> (200.8893, -199.9963)
  line L151 (200.8893, -199.9963) -> (199.6466, -204.3615)
  spline S165 degree 2 poles (199.6466, -204.3615) (199.4873, -204.935) (199.4873, -205.2111) knots 0 0 0 1 1 1
  spline S166 degree 2 poles (199.4873, -205.2111) (199.4873, -205.4342) (199.6891, -205.5722) knots 0 0 0 1 1 1
  spline S167 degree 2 poles (199.6891, -205.5722) (199.9971, -205.7634) (200.8574, -205.7634) knots 0 0 0 1 1 1
  spline S168 degree 2 poles (200.8574, -205.7634) (202.493, -205.7634) (205.3926, -204.3721) (206.5396, -202.9595) knots 0 0 0 1 2 2 2
  line L152 (206.5396, -202.9595) -> (206.9326, -202.9595)
  line L153 (206.9326, -202.9595) -> (205.5837, -206.5281)
  line L154 (205.5837, -206.5281) -> (194.5911, -206.5281)
  line L155 (194.5911, -206.5281) -> (194.7079, -206.1776)
  spline S169 degree 2 poles (194.7079, -206.1776) (195.6319, -206.1776) (196.4816, -205.4342) (196.8215, -204.1809) knots 0 0 0 1 2 2 2
  line L156 (196.8215, -204.1809) -> (199.2218, -195.801)
  spline S170 degree 2 poles (199.2218, -195.801) (199.4236, -195.1106) (199.4236, -194.707) knots 0 0 0 1 1 1
  spline S171 degree 2 poles (199.4236, -194.707) (199.4236, -194.3353) (198.8926, -193.9423) (197.9367, -193.8786) knots 0 0 0 1 2 2 2
  line L157 (197.9367, -193.8786) -> (198.0429, -193.5281)
  line L158 (198.0429, -193.5281) -> (208.5045, -193.5281)
  line L159 (208.5045, -193.5281) -> (207.6654, -196.7781)
  line L160 (207.6654, -196.7781) -> (207.3256, -196.7781)
  spline S172 degree 2 poles (207.3256, -196.7781) (207.2831, -195.8222) (207.0282, -195.4293) knots 0 0 0 1 1 1
  spline S173 degree 2 poles (207.0282, -195.4293) (206.614, -194.8132) (205.2651, -194.2503) (203.7569, -194.2503) knots 0 0 0 1 2 2 2
  line L161 (203.7569, -194.2503) -> (202.5249, -194.2503)
  line L162 (213.868, -200.1768) -> (212.7422, -204.1172)
  spline S174 degree 2 poles (212.7422, -204.1172) (212.4873, -204.9562) (212.4873, -205.3492) knots 0 0 0 1 1 1
  spline S175 degree 2 poles (212.4873, -205.3492) (212.4873, -205.7209) (213.0821, -206.1564) (214.0274, -206.1776) knots 0 0 0 1 2 2 2
  line L163 (214.0274, -206.1776) -> (213.8893, -206.5281)
  line L164 (213.8893, -206.5281) -> (207.6336, -206.5281)
  line L165 (207.6336, -206.5281) -> (207.7398, -206.1776)
  spline S176 degree 2 poles (207.7398, -206.1776) (208.685, -206.1776) (209.556, -205.4448) (209.9171, -204.1809) knots 0 0 0 1 2 2 2
  line L166 (209.9171, -204.1809) -> (212.3174, -195.8329)
  spline S177 degree 2 poles (212.3174, -195.8329) (212.5192, -195.1319) (212.5192, -194.7283) knots 0 0 0 1 1 1
  spline S178 degree 2 poles (212.5192, -194.7283) (212.5192, -194.3459) (212.02, -193.9423) (211.1066, -193.8786) knots 0 0 0 1 2 2 2
  line L167 (211.1066, -193.8786) -> (211.2022, -193.5281)
  line L168 (211.2022, -193.5281) -> (216.6082, -193.5281)
  spline S179 degree 2 poles (216.6082, -193.5281) (218.9236, -193.5281) (220.8035, -195.1319) (220.8035, -196.4064) knots 0 0 0 1 2 2 2
  spline S180 degree 2 poles (220.8035, -196.4064) (220.8035, -197.734) (219.6989, -198.8067) knots 0 0 0 1 1 1
  spline S181 degree 2 poles (219.6989, -198.8067) (219.0086, -199.4758) (217.2349, -199.9644) knots 0 0 0 1 1 1
  line L169 (217.2349, -199.9644) -> (218.3926, -203.9048)
  spline S182 degree 2 poles (218.3926, -203.9048) (218.8705, -205.4979) (219.5715, -206.1458) (220.3787, -206.1776) knots 0 0 0 1 2 2 2
  line L170 (220.3787, -206.1776) -> (220.3787, -206.5281)
  line L171 (220.3787, -206.5281) -> (216.3321, -206.5281)
  line L172 (216.3321, -206.5281) -> (214.5053, -200.1768)
  line L173 (214.5053, -200.1768) -> (214.1867, -200.1981)
  spline S183 degree 2 poles (214.1867, -200.1981) (214.0805, -200.1981) (213.868, -200.1768) knots 0 0 0 1 1 1
  spline S184 degree 2 poles (214.0274, -199.6033) (214.3566, -199.6245) (214.5796, -199.6245) knots 0 0 0 1 1 1
  spline S185 degree 2 poles (214.5796, -199.6245) (215.9604, -199.6245) (217.7447, -197.7021) (217.7447, -196.1515) knots 0 0 0 1 2 2 2
  spline S186 degree 2 poles (217.7447, -196.1515) (217.7447, -195.2275) (216.7888, -194.2716) (216.0135, -194.2716) knots 0 0 0 1 2 2 2
  spline S187 degree 2 poles (216.0135, -194.2716) (215.8223, -194.2716) (215.5568, -194.2822) knots 0 0 0 1 1 1
  line L174 (215.5568, -194.2822) -> (214.0274, -199.6033)
  point P0 (0, 0)
  dimension "d0" = 200
  dimension "d1" = 350
  constraints: 2 other
extrude "Extrusion17" add sketch "Sketch19" along normal blind 2
body "Solid1"
